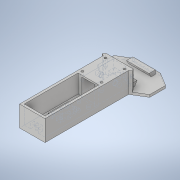
# Autodesk Inventor part: Griff_rechts
Saved by Autodesk Inventor 2021 (Build 250183000, 183)
## iProperties
Created: 2021-03-07
Part Number: Griff_rechts
Material: Generic
Document SubType Name: Modeling
Designer: Lukas
Density: 1 g/cm^3
Appearance: Default
Author: Lukas
Autodesk Inventor part; units mm, degrees
ref_plane "YZ Plane" through (0, 0, 0) normal (1, 0, 0) x (0, 1, 0)
ref_plane "XZ Plane" through (0, 0, 0) normal (0, 1, 0) x (-1, 0, 0)
ref_plane "XY Plane" through (0, 0, 0) normal (0, 0, 1) x (1, 0, 0)
sketch "Sketch27" plane through (0, 0, 0) normal (0, 1, 0) x (-1, 0, 0)
  line L0 (16, 72.5) -> (-16, 72.5)
  line L1 (-16, 72.5) -> (-16, -32.5)
  line L2 (16, -32.5) -> (16, 72.5)
  line L3 (16, -32.5) -> (32.5, -42.5)
  line L4 (32.5, -42.5) -> (32.5, -62.5)
  line L5 (32.5, -62.5) -> (16, -72.5)
  line L6 (16, -72.5) -> (-16, -72.5)
  line L7 (-16, -72.5) -> (-32.5, -62.5)
  line L8 (-32.5, -62.5) -> (-32.5, -42.5)
  line L9 (-32.5, -42.5) -> (-16, -32.5)
  circle A0 centre (0, -52.5) radius 1.6
  point P0 (0, 0)
  point P1 (0, -72.5)
  point P2 (0, 72.5)
  point P3 (-32.5, -52.5)
  dimension "d198" = 32
  dimension "d199" = 65
  dimension "d200" = 40
  dimension "d201" = 20
  dimension "d202" = 145
  dimension "d203" = 72.5
  dimension "d206" = 3.2
  constraints: 20 end point, 4 horizontal alignment, 4 vertical alignment, 3 midpoint, 3 perpendicular, 2 equal length, 1 centre point, 1 horizontal, 1 parallel, 1 vertical
  measures "d198" distance between parallel lines of L1 L2
  measures "d199" distance between parallel lines of L8 L4
  measures "d200" distance of L6.end L1.end
  measures "d201" distance of L7.end L8.end
  measures "d202" distance between parallel lines of L6 L0
  measures "d203" distance from line of point (0, 0) L0
  measures "d206" diameter of A0
extrude "Extrusion27" add sketch "Sketch27" along normal blind 3
sketch "Sketch28" plane through (0, 0, 0) normal (1, 0, 0) x (0, 1, 0)
  line L0 (3, -42.5) -> (3, -62.5) projected
  line L1 (3, -63) -> (8, -60)
  line L2 (8, -60) -> (8, -68)
  line L3 (0, -62.5) -> (0, -72.5) projected
  line L4 (8, -68) -> (3, -68)
  line L5 (3, -37) -> (8, -37)
  line L6 (8, -37) -> (8, -45)
  line L7 (8, -45) -> (3, -42)
  line L8 (3, -42) -> (3, -37)
  line L9 (3, -63) -> (3, -68)
  line L10 (3, -50.9) -> (3, -54.1) projected
  point P0 (0, 0)
  point P1 (3, -52.5)
  dimension "d207" = 15
  dimension "d208" = 21
  dimension "d209" = 8
  dimension "d210" = 7.5
  dimension "d211" = 5
  constraints: 16 end point, 8 point on line, 4 perpendicular, 2 equal length, 1 midpoint, 1 parallel
  measures "d207" distance of L6.end L1.end
  measures "d208" distance of L1.start L7.end
  measures "d209" distance of L1.end L2.end
  measures "d210" vertical distance of L1.end point (3, -52.5)
  measures "d211" horizontal distance of L1.start L1.end
extrude "Extrusion28" add sketch "Sketch28" along normal mid plane 28.25
sketch "Sketch29" plane through (0, 3, 0) normal (0, 1, 0) x (1, 0, 0)
  line L0 (-13, -69.5) -> (13, -69.5)
  line L1 (13, -69.5) -> (13, 37)
  line L2 (14.125, 37) -> (-14.125, 37) projected
  line L3 (-13, -69.5) -> (-13, 37)
  line L4 (14.125, 37) -> (17.125, 37)
  line L5 (17.125, 37) -> (18.8174, 34.2075)
  line L6 (16, 32.5) -> (32.5, 42.5) projected
  line L7 (-14.125, 37) -> (-17.125, 37)
  line L8 (-17.125, 37) -> (-18.8174, 34.2075)
  line L9 (-32.5, 42.5) -> (-16, 32.5) projected
  line L10 (-32.5, 42.5) -> (-16, 32.5) projected
  line L11 (16, -72.5) -> (16, 32.5) projected
  line L12 (-16, 32.5) -> (-16, -72.5) projected
  line L13 (-16, -72.5) -> (16, -72.5) projected
  point P0 (0, 0)
  dimension "d214" = 3
  dimension "d215" = 3
  dimension "d217" = 3
  dimension "d218" = 3
  constraints: 14 end point, 4 point on line, 3 horizontal, 3 perpendicular, 1 equal length, 1 vertical
  measures "d214" distance of L2.start L4.end
  measures "d215" distance between parallel lines of L11 L1
  measures "d217" distance between parallel lines of L12 L3
  measures "d218" distance between parallel lines of L13 L0
extrude "Extrusion29" add sketch "Sketch29" along normal blind 23 contours L0 L1 L2 L4 L5 L6 L11 L13 L12 L9 L8 L7 L3
sketch "Sketch33" plane through (0, 3, 0) normal (0, 1, 0) x (1, 0, 0)
  line L0 (8.1, 43.2) -> (-8.1, 43.2)
  line L1 (-8.1, 43.2) -> (-8.1, -2)
  line L2 (-8.1, -2) -> (8.1, -2)
  line L3 (8.1, -2) -> (8.1, 43.2)
  line L4 (-2.5, -17) -> (2.5, -17)
  line L5 (2.5, -17) -> (2.5, -35)
  line L6 (2.5, -35) -> (-2.5, -35)
  line L7 (-2.5, -35) -> (-2.5, -17)
  circle A0 centre (6, -8) radius 1.6
  circle A1 centre (-6, -8) radius 1.6
  point P0 (0, 0)
  point P1 (0, 43.2)
  point P2 (0, 43.2)
  point P3 (0, 43.2)
  point P4 (0, -17)
  dimension "d234" = 45.2
  dimension "d235" = 16.2
  dimension "d238" = 2
  dimension "d256" = 5
  dimension "d257" = 17
  dimension "d258" = 18
  dimension "d285" = 6
  dimension "d286" = 3.2
  dimension "d287" = 6
  dimension "d288" = 12
  constraints: 16 end point, 4 midpoint, 4 parallel, 2 centre point, 2 horizontal, 2 perpendicular, 2 vertical alignment, 1 equal radius, 1 horizontal alignment
  measures "d234" distance of L2.end L0.start
  measures "d235" distance of L1.end L2.end
  measures "d238" distance from line of L2 point (0, 0)
  measures "d256" distance of L4.start L4.end
  measures "d257" distance from line of point (0, 0) L4
  measures "d258" distance of L4.end L5.end
  measures "d285" distance from line of L2 A0.centre
  measures "d286" diameter of A0
  measures "d287" horizontal distance of A0.centre point (0, 0)
  measures "d288" distance of A1.centre A0.centre
extrude "Extrusion33" cut sketch "Sketch33" against normal through all both and the other way through all
chamfer "Chamfer5" distance 2.7 angle 45 4 edges at (8.1, 6.5, -43.2) (8.1, 1.5, -43.2) (-8.1, 1.5, -43.2) (-8.1, 6.5, -43.2)
sketch "Sketch34" plane through (8.1, 3, 2) normal (0, 0, -1) x (-1, 0, 0)
  line L0 (-4.9, 0) -> (-4.9, 23) projected
  line L1 (21.1, 0) -> (21.1, 23) projected
  line L2 (0, -3) -> (0, 0) projected
  line L3 (0, 0) -> (0, 21)
  line L4 (0, 0) -> (16.2, 0) projected
  line L5 (16.2, 0) -> (16.2, 21)
  line L6 (21.1, 0) -> (-4.9, 0) projected
  line L7 (-4.9, 23) -> (21.1, 23)
  line L8 (0, 21) -> (16.2, 21)
  point P0 (8.1, -3)
  dimension "d255" = 21
  constraints: 8 end point, 2 vertical, 1 horizontal
  measures "d255" distance of L2.end L3.end
extrude "Extrusion34" add sketch "Sketch34" along normal up to surface (39 mm away) contours L0 L7 L1 L6 L5 L8 L3
sketch "Sketch35" plane through (8.1, 0, -40.5) normal (-1, 0, 0) x (0, 0, 1)
  circle A0 centre (17.5, 13.5) radius 2.55
  line L0 (42.5, 0) -> (0, 0) projected
  line L1 (42.5, 0) -> (42.5, 3) projected
  circle A1 centre (17.5, 13.5) radius 2.75
  point P0 (40.5, 0)
  dimension "d247" = 13.5
  dimension "d248" = 5.1
  dimension "d249" = 25
  dimension "d252" = 5.5
  constraints: 2 centre point, 1 coincident
  measures "d247" distance from line of L0 A0.centre
  measures "d248" diameter of A0
  measures "d249" distance from line of A0.centre L1
  measures "d252" diameter of A1
extrude "Extrusion35" cut sketch "Sketch35" against normal blind 6 contours A0
extrude "Extrusion36" cut sketch "Sketch35" against normal blind 1
mirror "Mirror1" about plane through (0, 0, 0) normal (1, 0, 0) of "Extrusion35", "Extrusion36"
sketch "Sketch36" plane through (0, 3, 0) normal (0, 1, 0) x (1, 0, 0)
  line L0 (-2.5, -20) -> (-7.5, -20)
  line L1 (-7.5, -20) -> (-7.5, -45)
  line L2 (-7.5, -45) -> (-2.5, -45)
  line L3 (-2.5, -45) -> (-2.5, -20)
  line L4 (2.5, -45) -> (7.5, -45)
  line L5 (7.5, -45) -> (7.5, -20)
  line L6 (7.5, -20) -> (2.5, -20)
  line L7 (2.5, -20) -> (2.5, -45)
  circle A0 centre (-5, -24) radius 1.4
  circle A1 centre (-5, -41) radius 1.4
  circle A2 centre (5, -41) radius 1.4
  circle A3 centre (5, -24) radius 1.4
  point P0 (0, 0)
  point P1 (-2.5, -17)
  point P2 (2.5, -17)
  point P3 (5, -20)
  point P4 (-5, -20)
  dimension "d259" = 20
  dimension "d260" = 25
  dimension "d261" = 5
  dimension "d264" = 4
  dimension "d265" = 4
  dimension "d266" = 2.8
  constraints: 16 end point, 4 centre point, 4 parallel, 4 point on line, 4 vertical alignment, 3 equal radius, 2 horizontal, 2 horizontal alignment, 2 midpoint, 2 perpendicular, 1 collinear
  measures "d259" distance from line of point (0, 0) L0
  measures "d260" distance of L0.end L1.end
  measures "d261" distance of L0.start L0.end
  measures "d264" distance from line of L0 A0.centre
  measures "d265" distance from line of L2 A1.centre
  measures "d266" diameter of A0
extrude "Extrusion37" add sketch "Sketch36" along normal blind 3.5
sketch "Sketch41" plane through (0, 0, 0) normal (0, -1, 0) x (1, 0, 0)
  circle A0 centre (5, 31) radius 1.4
  circle A1 centre (-5, 31) radius 1.4
  line L0 (-2.5, 35) -> (2.5, 35) projected
  point P0 (0, 0)
  dimension "d296" = 5
  dimension "d297" = 10
  dimension "d298" = 2.8
  dimension "d299" = 4
  constraints: 2 centre point, 1 equal radius, 1 horizontal alignment
  measures "d296" horizontal distance of point (0, 0) A0.centre
  measures "d297" distance of A1.centre A0.centre
  measures "d298" diameter of A0
  measures "d299" distance from line of L0 A0.centre
extrude "Extrusion42" cut sketch "Sketch41" against normal through all
chamfer "Chamfer6" distance 3 angle 45 1 edges at (0, 3, 35)
sketch "Sketch42" plane through (0, 3, 0) normal (0, 1, 0) x (1, 0, 0)
  line L0 (-13, -69.5) -> (13, -69.5) projected
  line L1 (5, -69.5) -> (-5, -69.5)
  line L2 (-5, -69.5) -> (-5, -64.5)
  line L3 (-5, -64.5) -> (5, -64.5)
  line L4 (5, -64.5) -> (5, -69.5)
  circle A0 centre (0, -67) radius 1.4
  point P0 (0, 0)
  point P1 (0, -64.5)
  point P2 (0, -69.5)
  dimension "d305" = 5
  dimension "d306" = 10
  dimension "d307" = 2.8
  dimension "d308" = 2.5
  constraints: 8 end point, 2 midpoint, 2 parallel, 2 vertical alignment, 1 centre point, 1 horizontal, 1 perpendicular, 1 point on line
  measures "d305" distance of L3.end L1.start
  measures "d306" distance of L2.end L3.end
  measures "d307" diameter of A0
  measures "d308" distance from line of L3 A0.centre
extrude "Extrusion43" add sketch "Sketch42" along normal blind 6
sketch "Sketch43" plane through (0, 26, 0) normal (0, 1, 0) x (1, 0, 0)
  circle A0 centre (-12, 31.5) radius 1.4
  circle A1 centre (12, 31.5) radius 1.4
  circle A2 centre (-12, 2.5) radius 1.4
  circle A3 centre (12, 2.5) radius 1.4
  point P0 (0, 0)
  dimension "d314" = 2.8
  dimension "d315" = 12
  dimension "d316" = 24
  dimension "d317" = 2.5
  dimension "d318" = 31.5
  constraints: 4 centre point, 3 equal radius, 2 horizontal alignment, 2 vertical alignment
  measures "d314" diameter of A0
  measures "d315" horizontal distance of point (0, 0) A0.centre
  measures "d316" distance of A0.centre A1.centre
  measures "d317" vertical distance of point (0, 0) A3.centre
  measures "d318" vertical distance of A1.centre point (0, 0)
extrude "Extrusion44" cut sketch "Sketch43" against normal blind 10
body "Solid3"
